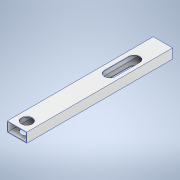
# Autodesk Inventor part: Frame
Saved by Autodesk Inventor 2020 (Build 240168000, 168)
## iProperties
Created: 2020-01-16
Part Number: Frame
Material: Aluminum 6061
Document SubType Name: Modeling
Designer: autum
Density: 2.7 g/cm^3
Appearance: Aluminum - Flat
Author: autum
Autodesk Inventor part; units mm, degrees
ref_plane "YZ Plane" through (0, 0, 0) normal (1, 0, 0) x (0, 1, 0)
ref_plane "XZ Plane" through (0, 0, 0) normal (0, 1, 0) x (-1, 0, 0)
ref_plane "XY Plane" through (0, 0, 0) normal (0, 0, 1) x (1, 0, 0)
sketch "Sketch1" plane through (0, 0, 0) normal (0, 0, 1) x (1, 0, 0)
  line L0 (-25.4, 12.7) -> (25.4, 12.7)
  line L1 (25.4, 12.7) -> (25.4, -12.7)
  line L2 (25.4, -12.7) -> (-25.4, -12.7)
  line L3 (-25.4, -12.7) -> (-25.4, 12.7)
  line L4 (-25.4, 12.7) -> (25.4, -12.7) construction
  line L5 (25.4, 12.7) -> (-25.4, -12.7) construction
  line L6 (-23.8125, 11.1125) -> (23.8125, 11.1125)
  line L7 (23.8125, 11.1125) -> (23.8125, -11.1125)
  line L8 (23.8125, -11.1125) -> (-23.8125, -11.1125)
  line L9 (-23.8125, -11.1125) -> (-23.8125, 11.1125)
  line L10 (-23.8125, 11.1125) -> (23.8125, -11.1125) construction
  line L11 (23.8125, 11.1125) -> (-23.8125, -11.1125) construction
  point P0 (0, 0)
  dimension "d0" = 50.8
  dimension "d1" = 25.4
  dimension "d2" = 47.625
  dimension "d3" = 22.225
  constraints: 24 end point, 4 midpoint, 4 parallel, 2 horizontal, 2 perpendicular
  measures "d0" distance of L1.end L2.end
  measures "d1" distance of L0.end L1.end
  measures "d2" distance of L7.end L8.end
  measures "d3" distance of L6.end L7.end
extrude "Extrusion1" add sketch "Sketch1" along normal blind 381
sketch "Sketch2" plane through (-25.4, 12.7, 0) normal (0, 1, 0) x (1, 0, 0)
  line L0 (0, 0) -> (0, -381) projected
  line L1 (50.8, -381) -> (0, -381) projected
  point P0 (25.4, 0)
  point P1 (25.4, -355.6)
  dimension "d13" = 25.4
  dimension "d14" = 25.4
  measures "d13" distance from line of L0 point (25.4, -355.6)
  measures "d14" distance from line of L1 point (25.4, -355.6)
hole "Hole1" at (0, 12.7, 355.6) direction (0, -1, 0) diameter 28.575 end through all
sketch "Sketch3" plane through (-25.4, 12.7, 0) normal (0, 1, 0) x (1, 0, 0)
  line L0 (40.972, -76.2) -> (40.972, -141.2421)
  arc A0 (40.972, -76.2) -> (12.397, -76.2) centre (26.6845, -76.2) ccw
  line L1 (12.397, -141.2421) -> (12.397, -76.2)
  arc A1 (12.397, -141.2421) -> (40.972, -141.2421) centre (26.6845, -139.7) ccw
  line L2 (50.8, 0) -> (0, 0) projected
  line L3 (50.8, -381) -> (0, -381) projected
  circle A2 centre (25.4, -355.6) radius 14.2875 projected
  point P0 (25.4, 0)
  dimension "d15" = 28.575
  dimension "d18" = 304.8
  dimension "d24" = 215.9
  dimension "d25" = 63.5
  constraints: 4 end point, 4 point on circle, 2 centre point, 1 tangent
  measures "d15" distance between parallel lines of L0 L1
  measures "d18" distance from line of L3 A0.centre
  measures "d24" vertical distance of A1.centre A2.centre
  measures "d25" distance of A0.centre A1.centre
extrude "Extrusion2" cut sketch "Sketch3" against normal through all contours L0 A1 L1 A0
body "Solid1"
